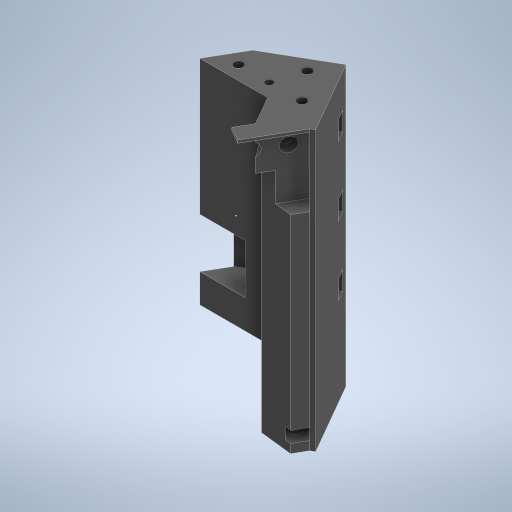
# Autodesk Inventor part: base_backwall_setter_upper
Saved by Autodesk Inventor 2024.1 (Build 281209000, 209)
## iProperties
Created: 2025-01-18
Part Number: base_backwall_setter_upper
Material: 一般
Document SubType Name: Modeling
Designer: hibik
Density: 1 g/cm^3
Appearance: 既定
Author: hibik
Autodesk Inventor part; units mm, degrees
ref_plane "YZ Plane" through (0, 0, 0) normal (1, 0, 0) x (0, 1, 0)
ref_plane "XZ Plane" through (0, 0, 0) normal (0, 1, 0) x (-1, 0, 0)
ref_plane "XY Plane" through (0, 0, 0) normal (0, 0, 1) x (1, 0, 0)
sketch "スケッチ2" plane through (0, 0, 0) normal (0, 1, 0) x (-1, 0, 0)
  line L0 (0, 0) -> (-8.6603, -15)
  line L1 (-8.6603, -15) -> (11.3397, -49.641)
  line L2 (48.1019, 0) -> (-18.1206, 0) projected
  line L3 (11.3397, -49.641) -> (5.9252, -52.7671) construction
  line L4 (0, 0) -> (-6.6711, 3.8516) construction
  line L5 (11.3397, -49.641) -> (24.3301, -42.141)
  line L6 (24.3301, -42.141) -> (0, 0)
  line L7 (0, 0) -> (8.2272, -4.75)
  line L8 (8.2272, -4.75) -> (-3.1754, -24.5)
  line L9 (-2.5935, -25.5079) -> (9.1002, -5.254)
  line L10 (9.1002, -5.254) -> (8.2272, -4.75)
  line L11 (-3.1754, -24.5) -> (2.5403, -27.8)
  line L12 (2.5403, -27.8) -> (12.2903, -10.9125)
  line L13 (12.2903, -10.9125) -> (6.5746, -7.6125)
  line L14 (6.5746, -7.6125) -> (-3.1754, -24.5)
  line L15 (11.3397, -49.641) -> (31.9282, -37.7543)
  line L16 (31.9282, -37.7543) -> (38.6416, -26.1264)
  line L17 (6.3397, -40.9808) -> (21.9282, -31.9808) construction
  line L18 (21.9282, -31.9808) -> (31.9282, -37.7543)
  line L19 (12.2903, -10.9125) -> (38.6416, -26.1264)
  line L20 (38.6416, -26.1264) -> (3.5066, -26.1264)
  line L21 (-2.3094, -23) -> (12.6388, -48.891)
  point P0 (9.2953, -16.1)
  point P1 (7.4475, -8.1165)
  point P2 (-2.3025, -25.004)
  point P3 (15.0841, -26.1264)
  point P4 (-1.7275, -24.0079)
  point P5 (-0.5774, -26)
  dimension "d11" = 60
  dimension "d12" = 60
  dimension "d13" = 40
  dimension "d15" = 15
  dimension "d16" = 9.5
  dimension "d17" = 1.0079
  dimension "d18" = 19.5
  dimension "d19" = 6.6
  dimension "d24" = 18
  dimension "d25" = 30
  dimension "d26" = 60
  dimension "d31" = 1.5
  constraints: 43 end point, 8 perpendicular, 6 point on line, 5 parallel, 4 collinear, 1 horizontal
  measures "d11" angle of L2 L0
  measures "d12" angle of L0 L1
  measures "d13" distance from line of L0.end L3
  measures "d15" distance between parallel lines of L1 L6
  measures "d16" distance between parallel lines of L0 L8
  measures "d17" distance between parallel lines of L8 L9
  measures "d18" distance between parallel lines of L11 L13
  measures "d19" distance between parallel lines of L14 L12
  measures "d24" distance from line of L17.end L1
  measures "d25" distance from line of L0.end L17
  measures "d26" angle of L17 L18
  measures "d31" distance between parallel lines of L1 L21
extrude "押し出し3" add sketch "スケッチ2" against normal blind 1 contours L9 L13 L12 L6 | L6 L12 L11 L21 L9 | L6 L20 L12 | L11 L12 L20 L6 L5 L21 | L20 L16 L15 L6
extrude "押し出し4" add sketch "スケッチ2" against normal blind 15 contours L6 L20 L12 | L11 L12 L20 L6 L5 L21 | L20 L16 L15 L6
sketch "スケッチ3" plane through (-9.2953, -15, -16.1) normal (0.8660254, 0, 0.5) x (0.5, 0, -0.8660254)
  circle A0 centre (8.51, 7.1) radius 1.25 projected
  circle A1 centre (-0.99, 7.1) radius 1.25 projected
  circle A2 centre (8.51, 7.1) radius 2.5
  circle A3 centre (-0.99, 7.1) radius 2.5
  point P0 (-9.2953, 15)
  dimension "d28" = 5
  constraints: 2 centre point, 2 coincident, 1 equal radius
  measures "d28" diameter of A2
extrude "押し出し5" cut sketch "スケッチ3" against normal blind 4 contours A0 | A1 | A2 | A3
sketch "スケッチ4" plane through (0, -15, 0) normal (0, -1, 0) x (1, 0, 0)
  point P0 (0, 0)
sketch "スケッチ5" plane through (0, -15, 0) normal (0, -1, 0) x (1, 0, 0)
  arc A0 (-18.3911, -20.4344) -> (-19.0567, -20.8273) centre (-17.2118, -23.1929) ccw projected
  arc A1 (-18.3911, -20.4344) -> (-13.9701, -14.9334) centre (-21.3392, -13.5382) ccw projected
  line L0 (-13.9701, -14.9334) -> (-12.1098, -5.108) projected
  line L1 (-12.1098, -5.108) -> (-7.7865, -8.3122) projected
  line L2 (-7.7865, -8.3122) -> (-2.7865, -16.9725) projected
  line L3 (-2.7865, -16.9725) -> (-7.1166, -19.4725) projected
  line L4 (-7.1166, -19.4725) -> (-19.0567, -20.8273) projected
  line L5 (-9.2953, -16.1) -> (-15.0841, -26.1264) projected
  line L6 (-15.0841, -26.1264) -> (-38.6416, -26.1264) projected
  line L7 (-38.6416, -26.1264) -> (-31.9282, -37.7543) projected
  line L8 (-31.9282, -37.7543) -> (-12.6388, -48.891) projected
  line L9 (-12.6388, -48.891) -> (0.5774, -26) projected
  line L10 (0.5774, -26) -> (-2.5403, -27.8) projected
  line L11 (-2.5403, -27.8) -> (-9.2953, -16.1) projected
  line L12 (-6.7887, -20.4417) -> (-12.1535, -21.0504)
  line L13 (-2.5403, -27.8) -> (-1.5011, -29.6)
  point P0 (0, 0)
  dimension "d32" = 1
  constraints: 4 end point, 3 point on line, 1 collinear, 1 parallel
  measures "d32" distance between parallel lines of L12 L4
extrude "押し出し6" add sketch "スケッチ5" along normal blind 10 contours L12 L11 L13 L9 L8 L7 L6 L5
sketch "スケッチ6" plane through (0, -25, 0) normal (0, -1, 0) x (1, 0, 0)
  line L0 (-7.4475, -8.1165) -> (1.7275, -24.0079) projected
  line L1 (1.7275, -24.0079) -> (-12.6388, -48.891) projected
  line L2 (-12.6388, -48.891) -> (-1.5011, -29.6) projected
  line L3 (-1.5011, -29.6) -> (-6.7887, -20.4417) projected
  line L4 (-6.7887, -20.4417) -> (-12.1535, -21.0504) projected
  line L5 (-12.1535, -21.0504) -> (-15.0841, -26.1264) projected
  line L6 (-15.0841, -26.1264) -> (-38.6416, -26.1264) projected
  line L7 (-38.6416, -26.1264) -> (-31.9282, -37.7543) projected
  line L8 (-31.9282, -37.7543) -> (-12.6388, -48.891) projected
  line L9 (-6.7887, -20.4417) -> (-0.7285, -19.754)
  line L10 (-6.7887, -20.4417) -> (-12.1535, -21.0504) projected
  point P0 (0, 0)
  constraints: 2 end point, 1 collinear, 1 point on line
ref_plane "作業平面1" through (-61.3397, -97, -49.641) normal (0, 1, 0) x (0, 0, 1)
extrude "押し出し7" add sketch "スケッチ6" along normal up to surface (72 mm away)
sketch "スケッチ7" plane through (-38.6416, -97, -26.1264) normal (0, -1, 0) x (1, 0, 0)
  circle A0 centre (18.1264, -8.3959) radius 1.5 projected
  circle A1 centre (18.1264, -8.3959) radius 12.5
  line L0 (18.1264, -8.3959) -> (34.2986, -8.3959)
  line L1 (40.369, 2.1184) -> (26.0028, -22.7646) projected
  circle A2 centre (17.3018, 12.5879) radius 1.5 projected
  circle A3 centre (18.1264, -8.3959) radius 1.5 projected
  line L2 (27.3018, -23.5146) -> (6.7134, -11.6279) projected
  line L3 (47.3018, 11.1264) -> (27.3018, -23.5146) projected
  line L4 (17.3018, 63.0879) -> (47.3018, 11.1264) projected
  line L5 (-22.6982, 63.0879) -> (17.3018, 63.0879) projected
  line L6 (-22.6982, 39.3144) -> (-22.6982, 63.0879) projected
  line L7 (6.7134, -11.6279) -> (-22.6982, 39.3144) projected
  line L8 (23.5575, 0) -> (0, 0) projected
  circle A4 centre (34.8109, 1.7454) radius 1.6 projected
  circle A5 centre (-18.6982, 58.0879) radius 1.6 projected
  circle A6 centre (-18.6982, 47.2241) radius 1.6 projected
  circle A7 centre (37.7217, 18.4196) radius 1.6 projected
  circle A8 centre (41.817, 11.3264) radius 1.6 projected
  circle A9 centre (-15.3681, 36.6183) radius 1.6 projected
  circle A10 centre (2.1319, 6.3074) radius 1.6 projected
  point P0 (38.6416, 26.1264)
  point P1 (30.6264, -8.3959)
  point P2 (8.8658, 0)
  dimension "d37" = 25
  constraints: 2 end point, 1 centre point, 1 coincident, 1 horizontal, 1 point on line
  measures "d37" diameter of A1
extrude "押し出し8" cut sketch "スケッチ7" against normal blind 50 contours A0 | A1 L2 L7 | L0 L1 L2 A1 | A1 L7 L8 picked at (15.3715, -13.9227)
fillet "フィレット1" radius 1 1 edges at (0.5774, -8, -26)
sketch "スケッチ9" plane through (-38.6416, -47, -26.1264) normal (0, -1, 0) x (1, 0, 0)
  arc A0 (12.138, -8.7682) -> (20.7982, -13.7682) centre (18.1264, -8.3959) ccw projected
  line L0 (20.7982, -13.7682) -> (24.1149, -8.0236) projected
  arc A1 (24.1149, -8.0236) -> (15.4546, -3.0236) centre (18.1264, -8.3959) ccw projected
  line L1 (15.0764, -13.6786) -> (4.3078, -7.4614)
  line L2 (21.1764, -3.1131) -> (15.7843, 0)
  line L3 (21.1264, -3.1997) -> (15.1264, -13.592) construction
  line L4 (23.5575, 0) -> (24.8091, 2.1678) projected
  line L5 (0, 0) -> (23.5575, 0) projected
  line L6 (6.7134, -11.6279) -> (0, 0) projected
  line L7 (26.0028, -22.7646) -> (6.7134, -11.6279) projected
  line L8 (34.2986, -8.3959) -> (26.0028, -22.7646) projected
  line L9 (30.6264, -8.3959) -> (34.2986, -8.3959) projected
  arc A2 (30.6264, -8.3959) -> (24.8091, 2.1678) centre (18.1264, -8.3959) ccw projected
  circle A3 centre (18.1264, -8.3959) radius 6.1
  line L10 (24.2165, -8.0476) -> (20.8698, -13.8442)
  point P0 (38.6416, 26.1264)
  point P1 (21.1764, -3.1131)
  dimension "d47" = 0.1
  dimension "d48" = 0.1
  constraints: 8 end point, 4 point on line, 2 parallel, 2 perpendicular, 2 point on circle, 2 tangent, 1 centre point, 1 coincident, 1 midpoint
  measures "d47" radial gap between concentric circles of A3 A0
  measures "d48" distance between parallel lines of L0 L10
ref_plane "作業平面2" through (-27.8453, -74.3, -42.2184) normal (0, 1, 0) x (0.5, 0, 0.8660254)
extrude "押し出し9" add sketch "スケッチ9" along normal up to surface (27.3 mm away) contours A3 L2 L5 L4 A2 L9 L8 L7 L6 L1 | L10 A3 picked at (22.361, -11.6675)
sketch "スケッチ10" plane through (-22.8572, -74.3, -26.1264) normal (0, -1, 0) x (1, 0, 0)
  line L0 (-11.4765, -7.4614) -> (-0.7079, -13.6786) projected
  line L1 (5.3921, -3.1131) -> (0, 0) projected
  line L2 (-15.7843, 0) -> (0, 0) projected
  line L3 (-11.4765, -7.4614) -> (-15.7843, 0) projected
  line L4 (-11.4765, -7.4614) -> (-9.071, -11.6279) projected
  line L5 (-9.071, -11.6279) -> (10.2185, -22.7646) projected
  line L6 (10.2185, -22.7646) -> (18.5143, -8.3959) projected
  line L7 (14.8421, -8.3959) -> (18.5143, -8.3959) projected
  arc A0 (14.8421, -8.3959) -> (9.0248, 2.1678) centre (2.3421, -8.3959) ccw projected
  line L8 (9.0248, 2.1678) -> (7.7732, 0) projected
  line L9 (7.7732, 0) -> (0, 0) projected
  line L10 (0, 0) -> (5.3921, -3.1131) projected
  arc A1 (8.4322, -8.0476) -> (5.3921, -3.1131) centre (2.3421, -8.3959) ccw projected
  line L11 (8.4322, -8.0476) -> (5.0855, -13.8442) projected
  arc A2 (-0.7079, -13.6786) -> (5.0855, -13.8442) centre (2.3421, -8.3959) ccw projected
  line L12 (-0.7079, -13.6786) -> (-11.4765, -7.4614) projected
  arc A3 (-0.7079, -13.6786) -> (5.0855, -13.8442) centre (2.3421, -8.3959) ccw projected
  line L13 (5.0855, -13.8442) -> (8.4322, -8.0476) projected
  arc A4 (8.4322, -8.0476) -> (5.3921, -3.1131) centre (2.3421, -8.3959) ccw projected
  circle A5 centre (2.3421, -8.3959) radius 6.1
  arc A6 (-0.7079, -13.6786) -> (5.0855, -13.8442) centre (2.3421, -8.3959) ccw projected
  line L14 (-0.4013, -2.9476) -> (-3.7479, -8.7442)
  point P0 (22.8572, 26.1264)
  dimension "d49" = 5.1
  dimension "d50" = 5.1
  constraints: 2 end point, 2 point on circle, 1 centre point, 1 coincident, 1 concentric, 1 parallel
  measures "d49" distance from line of A3.centre L13
  measures "d50" distance from line of L14 A3.centre
extrude "押し出し10" add sketch "スケッチ10" against normal blind 10 contours L3 L2 L1 A5 L0 | L0 A2 A5 A1 L1 L9 L8 A0 L7 L6 L5 L4 | L11 A5 | A5 L14
sketch "スケッチ12" plane through (0, 0, 0) normal (0, 1, 0) x (1, 0, 0)
  circle A0 centre (-8.1403, 31.0995) radius 1.6
  circle A1 centre (-16.201, 41.0609) radius 1.6
  line L0 (-9.7858, 33.9495) -> (-6.4949, 33.9495)
  line L1 (-6.4949, 33.9495) -> (-4.8494, 31.0995)
  line L2 (-4.8494, 31.0995) -> (-6.4949, 28.2495)
  line L3 (-6.4949, 28.2495) -> (-9.7858, 28.2495)
  line L4 (-9.7858, 28.2495) -> (-11.4312, 31.0995)
  line L5 (-11.4312, 31.0995) -> (-9.7858, 33.9495)
  line L6 (-19.051, 42.7063) -> (-16.201, 44.3518)
  line L7 (-16.201, 44.3518) -> (-13.351, 42.7063)
  line L8 (-13.351, 42.7063) -> (-13.351, 39.4154)
  line L9 (-13.351, 39.4154) -> (-16.201, 37.77)
  line L10 (-16.201, 37.77) -> (-19.051, 39.4154)
  line L11 (-19.051, 39.4154) -> (-19.051, 42.7063)
  line L12 (1.7275, 24.0079) -> (-12.6388, 48.891) projected
  line L13 (-12.6388, 48.891) -> (-31.9282, 37.7543) projected
  line L14 (-6.4949, 28.2495) -> (-2.1648, 30.7495)
  line L15 (-9.7858, 33.9495) -> (-5.4557, 36.4495)
  line L16 (-13.351, 42.7063) -> (-15.851, 47.0365)
  line L17 (-19.051, 39.4154) -> (-21.551, 43.7456)
  line L18 (-31.7134, 33.8264) -> (-28.4225, 33.8264)
  line L19 (-28.4225, 33.8264) -> (-26.777, 30.9764)
  line L20 (-26.777, 30.9764) -> (-28.4225, 28.1264)
  line L21 (-28.4225, 28.1264) -> (-31.7134, 28.1264)
  line L22 (-31.7134, 28.1264) -> (-33.3588, 30.9764)
  line L23 (-33.3588, 30.9764) -> (-31.7134, 33.8264)
  circle A2 centre (-30.0679, 30.9764) radius 1.6
  line L24 (-31.9282, 37.7543) -> (-38.6416, 26.1264) projected
  line L25 (-31.7134, 28.1264) -> (-36.0435, 30.6264)
  line L26 (-28.4225, 33.8264) -> (-32.7526, 36.3264)
  line L27 (-38.6416, 26.1264) -> (-15.0841, 26.1264) projected
  point P0 (0, 0)
  dimension "d51" = 3.2
  dimension "d52" = 5.7
  dimension "d53" = 5.7
  dimension "d54" = 5
  dimension "d55" = 5
  dimension "d56" = 7
  dimension "d75" = 5
  dimension "d76" = 2
  constraints: 48 end point, 7 perpendicular, 5 point on line, 3 centre point, 3 coincident, 3 parallel, 2 equal radius, 1 midpoint, 39 other
  measures "d51" diameter of A0
  measures "d52" distance between parallel lines of L5 L2
  measures "d53" distance between parallel lines of L11 L8
  measures "d54" distance from line of L12 A0.centre
  measures "d55" distance from line of L13 point (-16.201, 41.061)
  measures "d56" distance from line of L12 A1.centre
  measures "d75" distance from line of point (-30.068, 30.976) L24
  measures "d76" distance between parallel lines of L27 L21
extrude "押し出し12" cut sketch "スケッチ12" against normal blind 7 contours A0 | A1 | L15 L12 L14 L2 L1 L0 | L0 L1 L2 L3 L4 L5 | L11 L17 L13 L16 L7 L6 | L6 L7 L8 L9 L10 L11 | L23 L22 L25 L24 L26 L18 | L18 L19 L20 L21 L22 L23 | A2
extrude "押し出し13" add sketch "スケッチ12" against normal blind 3
extrude "押し出し14" cut sketch "スケッチ12" against normal blind 15 contours A0 | A1 | A2
sketch "スケッチ13" plane through (-8.0151, -97, -34.5223) normal (0, -1, 0) x (1, 0, 0)
  circle A0 centre (4.1845, 10.1413) radius 1.6
  line L0 (2.539, 12.9913) -> (5.8299, 12.9913)
  line L1 (5.8299, 12.9913) -> (7.4754, 10.1413)
  line L2 (7.4754, 10.1413) -> (5.8299, 7.2913)
  line L3 (5.8299, 7.2913) -> (2.539, 7.2913)
  line L4 (2.539, 7.2913) -> (0.8936, 10.1413)
  line L5 (0.8936, 10.1413) -> (2.539, 12.9913)
  line L6 (9.7426, 10.5143) -> (7.2866, 14.7683) projected
  line L7 (8.5146, 12.6413) -> (4.1845, 10.1413)
  line L8 (5.8299, 7.2913) -> (10.2263, 9.8296)
  line L9 (2.539, 12.9913) -> (6.8691, 15.4913)
  line L10 (3.6721, 0) -> (9.7426, 10.5143) projected
  line L11 (7.2866, 14.7683) -> (-4.1383, 13.4719) projected
  point P0 (8.0151, 34.5223)
  point P1 (8.9077, 9.0683)
  point P2 (5.2084, 14.5324)
  dimension "d63" = 3.2
  dimension "d64" = 5.7
  dimension "d65" = 5
  constraints: 18 end point, 3 perpendicular, 1 centre point, 1 coincident, 1 midpoint, 1 parallel, 1 point on line, 13 other
  measures "d63" diameter of A0
  measures "d64" distance between parallel lines of L5 L2
  measures "d65" distance from line of L6 A0.centre
extrude "押し出し15" cut sketch "スケッチ13" against normal blind 7 contours A0 | L9 L11 L6 L7 L1 L0 | L0 L1 L2 L3 L4 L5 | L7 L6 L10 L8 L2 L1
extrude "押し出し16" add sketch "スケッチ13" against normal blind 3
extrude "押し出し17" cut sketch "スケッチ13" against normal blind 15 contours A0
sketch "スケッチ14" plane through (-1.5011, -25, -29.6) normal (0.8660254, 0, -0.5) x (-0.5, 0, -0.8660254)
  line L0 (22.2753, 25) -> (-6.4571, 25)
  line L1 (-6.4571, 25) -> (-6.4571, -72)
  line L2 (-6.4571, -72) -> (22.2753, -72)
  line L3 (22.2753, -72) -> (22.2753, 25)
  line L4 (5.6838, -72) -> (-6.4571, -72) projected
  line L5 (-6.4571, 0) -> (-6.4571, -65) projected
  point P0 (-26.3849, 25)
  constraints: 8 end point, 2 collinear, 2 parallel, 1 horizontal, 1 perpendicular
extrude "押し出し18" add sketch "スケッチ14" along normal blind 1.5
sketch "スケッチ15" plane through (0, 0, 0) normal (0, 1, 0) x (1, 0, 0)
  circle A0 centre (-19.3806, 30.9764) radius 1.6 projected
  circle A1 centre (-19.3806, 30.9764) radius 1.35
  point P0 (0, 0)
  dimension "d77" = 2.7
  constraints: 1 centre point, 1 coincident
  measures "d77" diameter of A1
extrude "押し出し19" cut sketch "スケッチ15" against normal blind 15 contours A1
sketch "スケッチ16" plane through (-31.9282, -74.3, -37.7543) normal (-0.5, 0, -0.8660254) x (-0.8660254, 0, 0.5)
  line L0 (-18.7735, 56.0091) -> (-21.6235, 57.6546)
  line L1 (-21.6235, 57.6546) -> (-21.6235, 60.9454)
  line L2 (-21.6235, 60.9454) -> (-18.7735, 62.5909)
  line L3 (-18.7735, 62.5909) -> (-15.9235, 60.9454)
  line L4 (-15.9235, 60.9454) -> (-15.9235, 57.6546)
  line L5 (-15.9235, 57.6546) -> (-18.7735, 56.0091)
  line L6 (-23.7735, -22.7) -> (-23.7735, 74.3) projected
  line L7 (-18.7735, 62.5909) -> (-23.7735, 62.5909)
  line L8 (-18.7735, 56.0091) -> (-23.7735, 56.0091)
  line L9 (-23.7735, 74.3) -> (0, 74.3) projected
  circle A0 centre (-18.7735, 59.3) radius 1.6
  point P0 (-8.7735, 74.3)
  dimension "d80" = 5.7
  dimension "d81" = 5
  dimension "d82" = 15
  dimension "d83" = 3.2
  constraints: 16 end point, 2 perpendicular, 2 point on line, 1 centre point, 1 coincident, 1 parallel, 13 other
  measures "d80" distance between parallel lines of L0 L3
  measures "d81" distance from line of L6 point (-18.774, 59.3)
  measures "d82" distance from line of L9 point (-18.774, 59.3)
  measures "d83" diameter of A0
extrude "押し出し20" cut sketch "スケッチ16" against normal blind 7 contours L8 L6 L7 L2 L1 L0 | L0 L1 L2 L3 L4 L5 | A0
extrude "押し出し21" add sketch "スケッチ16" against normal blind 3
extrude "押し出し22" cut sketch "スケッチ16" against normal blind 16 contours A0
pattern_linear "矩形状パターン1" count 3 spacing 24 along (0, -1, 0) of "押し出し20", "押し出し21", "押し出し22"
equation "\"d50\" = d49"
equation "\"d75\" = d55"
